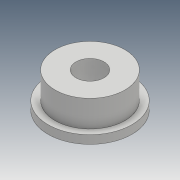
# Autodesk Inventor part: rotating_finger-bearing
Saved by Autodesk Inventor 2018 (Build 220112000, 112)
## iProperties
Created: 2019-04-02
Part Number: rotating_finger-bearing
Material: Generic
Document SubType Name: Modeling
Designer: Tsche
Density: 1 g/cm^3
Appearance: Default
Author: Tsche
Autodesk Inventor part; units mm, degrees
ref_plane "YZ Plane" through (0, 0, 0) normal (1, 0, 0) x (0, 1, 0)
ref_plane "XZ Plane" through (0, 0, 0) normal (0, 1, 0) x (-1, 0, 0)
ref_plane "XY Plane" through (0, 0, 0) normal (0, 0, 1) x (1, 0, 0)
sketch "Sketch1" plane through (0, 0, 0) normal (0, 1, 0) x (-1, 0, 0)
  line L0 (0, 0) -> (0, 7.0304)
  line L1 (-1, 0) -> (-3, 0)
  line L2 (-3, 0) -> (-3, 0.6)
  line L3 (-3, 0.6) -> (-2.5, 0.6)
  line L4 (-2.5, 0.6) -> (-2.5, 2.5)
  line L5 (-2.5, 2.5) -> (-1, 2.5)
  line L6 (-1, 0) -> (-1, 2.5)
  dimension "d0" = 5
  dimension "d1" = 0.6
  dimension "d2" = 2.5
  dimension "d3" = 6
  dimension "d5" = 2
  constraints: 14 end point, 4 perpendicular, 2 vertical, 1 horizontal, 1 point on line
  measures "d0" diameter of L4 L0
  measures "d1" distance of L1.end L2.end
  measures "d2" distance between parallel lines of L5 L1
  measures "d3" diameter of L2 L0
  measures "d5" diameter of L6 L0
revolve "Revolution1" add sketch "Sketch1" angle 360 about axis through (0, 0, 0) along (0, 0, 1)
body "Solid1"
